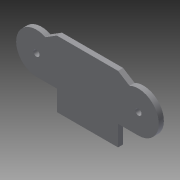
# Autodesk Inventor part: support_puissance
Saved by Autodesk Inventor 2014 SP1 (Build 180222100, 222)
## iProperties
Created: 2015-02-02
Part Number: support_puissance
Material: Générique
Document SubType Name: Modeling
Designer: astralien3000
Density: 1 g/cm^3
Appearance: Par défaut
Author: astralien3000
Autodesk Inventor part; units mm, degrees
ref_plane "YZ Plane" through (0, 0, 0) normal (1, 0, 0) x (0, 1, 0)
ref_plane "XZ Plane" through (0, 0, 0) normal (0, 1, 0) x (-1, 0, 0)
ref_plane "XY Plane" through (0, 0, 0) normal (0, 0, 1) x (1, 0, 0)
sketch "Esquisse1" plane through (0, 0, 0) normal (0, 1, 0) x (-1, 0, 0)
  line L0 (-30, 25) -> (30, 25)
  line L1 (30, 25) -> (30, -40)
  line L2 (30, -40) -> (-30, -40)
  line L3 (-30, -40) -> (-30, 25)
  line L4 (-30, 25) -> (-70, 25) construction
  line L5 (-70, 25) -> (-70, 0) construction
  line L6 (-70, 0) -> (-30, 0) construction
  line L7 (-30, 0) -> (-30, 25) construction
  line L8 (30, 25) -> (70, 25) construction
  line L9 (70, 25) -> (70, 0) construction
  line L10 (70, 0) -> (30, 0) construction
  line L11 (30, 0) -> (30, 25) construction
  line L12 (-50, 0) -> (50, 0) construction
  line L13 (50, 0) -> (50, -40) construction
  line L14 (50, -40) -> (-50, -40) construction
  line L15 (-50, -40) -> (-50, 0) construction
  circle A0 centre (-50, 0) radius 20
  circle A1 centre (50, 0) radius 20
  line L16 (-70, 0) -> (-30, 25)
  line L17 (70, 0) -> (30, 25)
  line L18 (50, -20) -> (-50, -20)
  line L19 (-70, 0) -> (-50, -20)
  line L20 (50, -20) -> (70, 0)
  point P0 (0, 0)
  dimension "d8" = 40
  dimension "d9" = 40
  dimension "d0" = 25
  dimension "d1" = 140
  dimension "d2" = 60
  dimension "d3" = 65
  dimension "d4" = 30
  dimension "d5" = 25
  dimension "d6" = 100
  dimension "d7" = 50
  dimension "d10" = 70
  constraints: 42 end point, 8 parallel, 4 horizontal, 4 perpendicular, 3 midpoint, 2 coincident, 2 vertical alignment, 1 collinear, 4 other
  measures "d0" distance between parallel lines of L4 L6
  measures "d1" distance between parallel lines of L9 L5
  measures "d2" distance of L0.start L0.end
  measures "d3" distance of L0.end L1.end
  measures "d4" distance from line of point (0, 0) L1
  measures "d5" distance from line of point (0, 0) L0
  measures "d6" distance between parallel lines of L13 L15
  measures "d7" distance from line of point (0, 0) L15
  measures "d10" distance from line of point (0, 0) L9
extrude "Extrusion1" add sketch "Esquisse1" along normal blind 5
sketch "Esquisse2" plane through (0, 5, 0) normal (0, 1, 0) x (1, 0, 0)
  arc A0 (41.236, -17.9775) -> (50, 20) centre (50, 0) ccw projected
  arc A1 (-50, 20) -> (-41.236, -17.9775) centre (-50, 0) ccw projected
  circle A2 centre (-50, 0) radius 3
  circle A3 centre (50, 0) radius 3
  point P0 (0, 0)
  dimension "d13" = 6
  dimension "d14" = 6
  constraints: 2 centre point, 2 coincident
  measures "d13" diameter of A2
  measures "d14" diameter of A3
extrude "Extrusion2" cut sketch "Esquisse2" against normal through all
sketch "Esquisse3" plane through (0, 5, 0) normal (0, 1, 0) x (1, 0, 0)
  circle A0 centre (-50, 0) radius 3 projected
  circle A1 centre (50, 0) radius 3 projected
  line L0 (30, 40) -> (-30, 40) projected
  arc A2 (-50, 20) -> (-41.236, -17.9775) centre (-50, 0) ccw projected
  line L1 (0, 0) -> (0, 40) construction
  line L2 (-50, 0) -> (-50, 20) construction
  circle A3 centre (-50, 0) radius 15 construction
  circle A4 centre (-50, 15) radius 4.5
  circle A5 centre (50, 15) radius 4.5
  circle A6 centre (-60.6066, 10.6066) radius 4.5
  circle A7 centre (-65, 0) radius 4.5
  circle A8 centre (-60.6066, -10.6066) radius 4.5
  circle A9 centre (-50, -15) radius 4.5
  circle A10 centre (-39.3934, -10.6066) radius 4.5
  circle A11 centre (-35, 0) radius 4.5
  circle A12 centre (-39.3934, 10.6066) radius 4.5
  circle A13 centre (39.3934, 10.6066) radius 4.5
  circle A14 centre (35, 0) radius 4.5
  circle A15 centre (39.3934, -10.6066) radius 4.5
  circle A16 centre (50, -15) radius 4.5
  circle A17 centre (60.6066, -10.6066) radius 4.5
  circle A18 centre (65, 0) radius 4.5
  circle A19 centre (60.6066, 10.6066) radius 4.5
  dimension "d17" = 30
  dimension "d18" = 9
  dimension "d21" = 360
  dimension "d25" = 360
  constraints: 16 centre point, 4 end point, 1 coincident, 1 midpoint, 1 point on line, 1 symmetric about line, 1 vertical alignment, 37 other
  measures "d18" diameter of A4
extrude "Extrusion3" cut sketch "Esquisse3" against normal blind 2.5 contours A4 | A5 | A6 | A7 | A8 | A9 | A10 | A11 | A12 | A13 | A14 | A15 | A16 | A17 | A18 | A19
equation "\"d9\" = d8"
equation "\"d4\" = 0.5 * d2"
equation "\"d5\" = d0"
equation "\"d7\" = 0.5 * d6"
equation "\"d10\" = 0.5 * d1"
equation "\"d14\" = d13"
